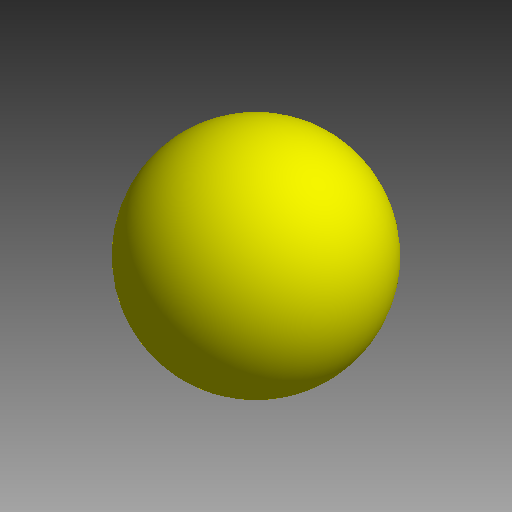
# Autodesk Inventor part: W 61705-2RZ_PART3
Saved by Autodesk Inventor 2018 (Build 220112000, 112)
## iProperties
Category: PARTsolutions
Company: SKF
Part Number: W 61705-2RZ_PART3
Material: Stainless Steel
Catalog Web Link: www.cadenas.de
Description: -Deep groove ball bearings
Vendor: SKF
Document SubType Name: Modeling
Designer: partserver
Manufacturer: SKF
Mass: 0.0167741 g
Surface Area: 0.0792229 cm^2
Volume: 0.00209677 cm^3
Density: 8 g/cm^3
Appearance: Semi-Polished
PSOL_IDENT_0: {$CADENAS_DATA\23d-libs\skf\bearings_units_and_housings\ball_bearings\deep_groove_ball_bearings\bb1_
PSOL_IDENT_1: 001_101.prj},201 {VTYP=3D},{NB=W 61705-2RZ_PART3},{LINA=W 61705-2RZ_PART3},{NN=BB1_001_101_PART3},{N
PSOL_IDENT_2: OPRJ=TRUE},{DATE=19.12.2019 14:34:47},{GEOMDATE=18.12.2019 13:53:11},{VERSION=},{LINEID=17800},{WBVA
PSOL_IDENT_3: R=},{WBNUMERIC=}  {NB=W 61705-2RZ_PART3},{LINA=W 61705-2RZ_PART3},{KT=DUMMY},{PRODUCTID=},{DESIGNATI
PSOL_IDENT_4: ON=W 61705-2RZ},{DD=25.000},{D=32.000},{B=4.000},{C=0.000},{DD1=27.27},{DD2=0.00},{D1=0.00},{D2=30.2
PSOL_IDENT_5: 9},{D3=0.000},{D4=0.000},{HH=MIN},{BB=0.000},{FF=0.00},{R0MAX=MIN},{R0=MIN},{R12=0.20},{PITCH=28.50}
PSOL_IDENT_6: ,{DW=1.588},{DDAMIN=26.500},{DDAMAX=27.000},{DDBMIN=MIN},{DDBMAX=MIN},{DBMIN=MIN},{DAMAX=30.500},{BB
PSOL_IDENT_7: AMIN=MIN},{CAMAX=MIN},{RAMAX=0.200},{LOAD1=0.618},{LOAD2=0.465},{LOAD3=0.020},{SPEED1=43000},{SPEED2=
PSOL_IDENT_8: 20000},{KR=0.015},{F0=8.800},{Z=21},{II=1},{MASS=0.007},{BEARING=W 61705-2RZ},{RING=},{HELP=1.218},{
PSOL_IDENT_9: HELP2=0.855},{DD1ALG=13.635},{YALG=13.635},{PITCH1=28.500},{DW1=1.588},{YALG1=14.782},{HALG1=1.218},
PSOL_IDENT_10: {SH=13.635},{CU=0.482},{DESIGN=dgbb2rs},{HALG=1.135},{B1=0},{SHIELDHELP=2}
NB: W 61705-2RZ_PART3
NT: Deep groove ball bearings
NBSYN: $DESIGNATION._PART3
LINA: W 61705-2RZ_PART3
CATALOG: SKF
SUPPLIER: SKF
ARTICLENO: W 61705-2RZ_PART3
BOMINFO: W 61705-2RZ_PART3
CREATOR: CADENAS GmbH
Title: W 61705-2RZ_PART3
Author: Cadenas PARTsolutions
Comments: Deep groove ball bearings
Autodesk Inventor part; units mm, degrees
ref_plane "YZ Plane" through (0, 0, 0) normal (1, 0, 0) x (0, 1, 0)
ref_plane "XZ Plane" through (0, 0, 0) normal (0, 1, 0) x (-1, 0, 0)
ref_plane "XY Plane" through (0, 0, 0) normal (0, 0, 1) x (1, 0, 0)
sketch "Sketch_6" plane through (0, 0, 0) normal (0, 0, 1) x (1, 0, 0)
  line L0 (2.794, 14.25) -> (1.206, 14.25)
  arc A0 (2.794, 14.25) -> (1.206, 14.25) centre (2, 14.25) ccw
  line L1 (2.794, 14.25) -> (1.206, 14.25)
  dimension "d0" = 360
  constraints: 4 end point, 2 point on circle, 1 centre point
revolve "Revolution1" add sketch "Sketch_6" angle 360 about axis through (2.794, 14.25, 0) along (1, 0, 0)
body "Solid1"
